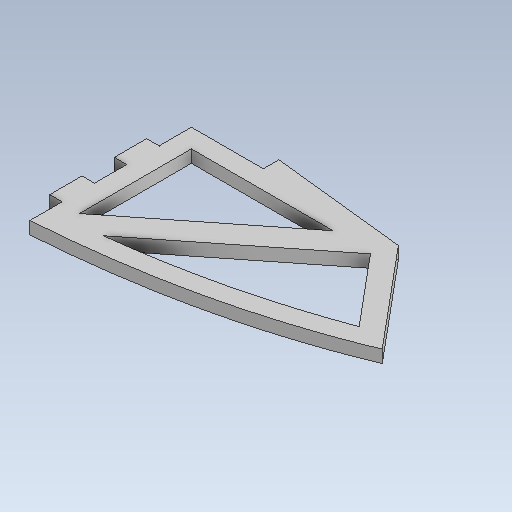
# Autodesk Inventor part: bulkhead_F2
Saved by Autodesk Inventor 2020.3 (Build 243373000, 373)
## iProperties
Created: 2020-05-22
Part Number: bulkhead_F2
Material: Generic
Document SubType Name: Modeling
Designer: kardo
Density: 1 g/cm^3
Appearance: Default
Mass: 0.941689 g
Surface Area: 14.623 cm^2
Volume: 0.941689 cm^3
Author: kardo
Autodesk Inventor part; units mm, degrees
ref_plane "YZ Plane" through (0, 0, 0) normal (1, 0, 0) x (0, 1, 0)
ref_plane "XZ Plane" through (0, 0, 0) normal (0, 1, 0) x (-1, 0, 0)
ref_plane "XY Plane" through (0, 0, 0) normal (0, 0, 1) x (1, 0, 0)
derived "base_sketch.ipt"
sketch "bulkhead_F2" plane through (0, 158.1, 33.6972) normal (0, 1, 0) x (-1, 0, 0)
  line L0 (19.176, 13.1208) -> (62.322, 13.1208)
  line L1 (62.322, 13.1208) -> (62.322, -20.1682)
  line L2 (0, -33.6972) -> (-11.5056, -33.6972)
  line L3 (-11.5056, -36.1839) -> (-34.5168, -33.6972)
  line L4 (-11.5056, -33.6972) -> (-11.5056, -36.1839)
  line L5 (-34.5168, -33.6972) -> (-57.528, -6.1572)
  line L6 (0, 5.8272) -> (0, -20.0113)
  line L7 (0, -20.0113) -> (-11.5056, -20.0113)
  line L8 (-11.5056, -20.0113) -> (-11.5056, -22.4981)
  line L9 (-11.5056, -22.4981) -> (-32.9405, -20.1817)
  line L10 (-32.9405, -20.1817) -> (-46.0224, -4.5252)
  line L11 (-57.528, -9.9639) -> (-57.528, -6.1572) construction
  line L12 (-38.352, 3.0228) -> (-38.352, -1.6402) construction
  line L13 (-19.176, 8.898) -> (-19.176, 3.3852) construction
  line L14 (0, 12.2028) -> (0, 5.8272) construction
  spline S0 degree 4 poles (-57.528, -6.1572) (-46.0483, 0.508) (-30.6129, 6.8309) (-11.2214, 11.3442) (8.3201, 13.1208) (15.5662, 13.1208) (19.176, 13.1208) knots 0 0 0 0 0 0.630279 0.815816 1 1 1 1 1
  spline S1 degree 3 poles (-57.528, -9.9639) (-39.1077, -0.0881) (-19.5511, 4.4627) (0, 5.8272) knots 0 0 0 0 1 1 1 1
  line L15 (0, 2.0028) -> (-57.528, -6.1572) construction
  line L16 (0, 19.4965) -> (0, 13.1208) construction
  line L17 (0, 13.1208) -> (-57.528, 13.1208) construction
  line L18 (-57.528, 13.1208) -> (-57.528, 16.9276) construction
  line L19 (-57.528, 16.9276) -> (0, 19.4965) construction
  line L20 (-38.352, 17.7839) -> (-38.352, 13.1208) construction
  line L21 (-19.176, 18.6402) -> (-19.176, 13.1208) construction
  line L22 (-46.0224, -4.5252) -> (-46.0224, -0.2046) construction
  line L23 (-46.0224, 17.4414) -> (-46.0224, 13.1208) construction
ref_plane "bulkhead_F2_plane" through (0, 158.1, 33.6972) normal (0, 1, 0) x (-1, 0, 0)
sketch "Sketch2" plane through (0, 158.1, 33.6972) normal (0, 1, 0) x (-1, 0, 0)
  spline S0 degree 3 poles (-57.528, -9.9639) (-39.1077, -0.0881) (-19.5511, 4.4627) (0, 5.8272) knots 0 0 0 0 1 1 1 1 projected
  line L0 (-32.9405, -20.1817) -> (-46.0224, -4.5252) projected
  line L1 (-11.5056, -22.4981) -> (-32.9405, -20.1817) projected
  line L2 (-11.5056, -20.0113) -> (-11.5056, -22.4981) projected
  line L3 (0, -20.0113) -> (-11.5056, -20.0113) projected
  line L4 (-41.0539, -5.7927) -> (-31.8679, -16.7866)
  line L5 (-31.8679, -16.7866) -> (-7.9914, 2.0657)
  line L6 (-32.9405, -20.1817) -> (0, 5.8272) construction
  line L7 (-25.6978, -17.0113) -> (-3, -17.0113)
  line L8 (-3, -17.0113) -> (-3, 0.9102)
  line L9 (-3, 0.9102) -> (-25.6978, -17.0113)
  line L10 (0, 0.6595) -> (2, 0.6595)
  line L11 (2, 0.6595) -> (2, -4.5082)
  line L12 (2, -4.5082) -> (0, -4.5082)
  line L13 (0, -9.6759) -> (2, -9.6759)
  line L14 (2, -9.6759) -> (2, -14.8436)
  line L15 (2, -14.8436) -> (0, -14.8436)
  spline S1 degree 2 poles (-41.0539, -5.7927) (-24.9977, 0.1352) (-7.9914, 2.0657) knots 0 0 0 1 1 1
  line L16 (-41.0539, -5.7927) -> (-42.1074, -2.9838) construction
  line L17 (-24.7602, -0.8642) -> (-25.4464, 2.0563) construction
  line L18 (-7.9914, 2.0657) -> (-8.3445, 5.0448) construction
  line L19 (-41.0539, -5.7927) -> (-24.7602, -0.8642) construction
  line L20 (-24.7602, -0.8642) -> (-7.9914, 2.0657) construction
  line L21 (0, 0.6595) -> (0, 5.8272)
  line L22 (0, -4.5082) -> (0, -9.6759)
  line L23 (0, -14.8436) -> (0, -20.0113)
  point P0 (0, -33.6972)
  dimension "d1" = 4
  dimension "d2" = 3
  dimension "d4" = 3
  dimension "d5" = 3
  dimension "d6" = 2
  dimension "d7" = 3
  constraints: 40 end point, 7 equal length, 4 collinear, 4 horizontal, 4 parallel, 2 vertical, 10 other
  measures "d1" distance between parallel lines of L9 L5
  measures "d2" distance between parallel lines of L3 L7
  measures "d4" distance between parallel lines of L0 L4
  measures "d5" distance of L4.start L16.end
  measures "d6" distance of L14.end L15.end
  measures "d7" distance between parallel lines of L22 L8
extrude "Extrusion1" add sketch "Sketch2" along normal blind 2
equation "\"d6\" = stringer_thickness"
equation "\"d8\" = bulkhead_thickness"
equation "\"stringer_thickness\" = 2"
equation "\"bulkhead_thickness\" = 2"
body "Solid1"
